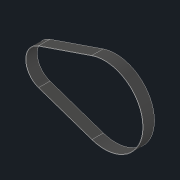
# Autodesk Inventor part: belt5
Saved by Autodesk Inventor 2021 (Build 250183000, 183)
## iProperties
Created: 2021-08-06
Part Number: belt5
Material: ゴム
Document SubType Name: Modeling
Designer: yuta0
Density: 0.93 g/cm^3
Appearance: ゴム - 黒
購入先: ミスミ
在庫数: 0.0
Author: yuta0
Autodesk Inventor part; units mm, degrees
ref_plane "YZ Plane" through (0, 0, 0) normal (1, 0, 0) x (0, 1, 0)
ref_plane "XZ Plane" through (0, 0, 0) normal (0, 1, 0) x (-1, 0, 0)
ref_plane "XY Plane" through (0, 0, 0) normal (0, 0, 1) x (1, 0, 0)
sketch "スケッチ1" plane through (0, 0, 0) normal (0, 0, 1) x (1, 0, 0)
  arc A0 (-5.5746, 16.2597) -> (-5.5746, -16.2597) centre (0, 0) ccw
  arc A1 (41.8508, -32.5193) -> (41.8508, 32.5193) centre (53, 0) ccw
  line L0 (-5.5746, 16.2597) -> (41.8508, 32.5193)
  line L1 (-5.5746, -16.2597) -> (41.8508, -32.5193)
  line L2 (41.715, 32.9157) -> (-5.7105, 16.656)
  arc A2 (-5.7105, 16.656) -> (-5.7105, -16.656) centre (0, 0) ccw
  line L3 (-5.7105, -16.656) -> (41.715, -32.9157)
  arc A3 (41.715, -32.9157) -> (41.715, 32.9157) centre (53, 0) ccw
  line L4 (41.9744, 32.1589) -> (-5.451, 15.8993)
  arc A4 (-5.451, 15.8993) -> (-5.451, -15.8993) centre (0, 0) ccw
  line L5 (-5.451, -15.8993) -> (41.9744, -32.1589)
  arc A5 (41.9744, -32.1589) -> (41.9744, 32.1589) centre (53, 0) ccw
  dimension "d6" = 34.3775
  dimension "d7" = 68.7549
  dimension "d8" = 53
  dimension "d11" = 0.419
  dimension "d12" = 0.8
  constraints: 12 end point, 12 point on circle, 6 centre point, 4 tangent, 1 coincident, 1 horizontal alignment, 6 other
  measures "d6" diameter of A0
  measures "d7" diameter of A1
  measures "d8" distance of A1.centre A0.centre
  measures "d11" distance between parallel lines of L0 L2
  measures "d12" distance between parallel lines of L2 L4
extrude "押し出し1" add sketch "スケッチ1" along normal mid plane 10 contours L0 A1 L1 A0
